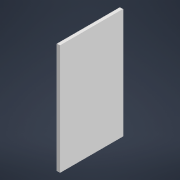
# Autodesk Inventor part: TorraumSeiteBalleinwurf
Saved by Autodesk Inventor 2021.4 (Build 254397000, 397)
## iProperties
Created: 2022-02-22
Part Number: TorraumSeiteBalleinwurf
Material: Generisch
Document SubType Name: Modeling
Designer: valen
Density: 1 g/cm^3
Appearance: Vorgabe
Author: valen
Autodesk Inventor part; units mm, degrees
ref_plane "YZ Plane" through (0, 0, 0) normal (1, 0, 0) x (0, 1, 0)
ref_plane "XZ Plane" through (0, 0, 0) normal (0, 1, 0) x (-1, 0, 0)
ref_plane "XY Plane" through (0, 0, 0) normal (0, 0, 1) x (1, 0, 0)
sketch "Skizze1" plane through (0, 0, 0) normal (1, 0, 0) x (0, 1, 0)
  line L0 (0, 0) -> (132, 0)
  line L1 (132, 0) -> (132, -80)
  line L2 (132, -80) -> (0, -80)
  line L3 (0, -80) -> (0, 0)
  dimension "d0" = 80
  dimension "d1" = 132
  constraints: 8 end point, 2 parallel, 1 horizontal, 1 perpendicular
  measures "d0" distance between parallel lines of L2 L0
  measures "d1" distance between parallel lines of L1 L3
extrude "Extrusion1" add sketch "Skizze1" along normal blind 4
sketch "Sketch2" plane through (0, 0, 0) normal (1, 0, 0) x (0, 1, 0)
  line L0 (0, 0) -> (0, -80) projected
  line L1 (0, 0) -> (-8, 0)
  line L2 (-8, 0) -> (-8, -80)
  line L3 (-8, -80) -> (0, -80)
  line L4 (0, -80) -> (0, 0)
  line L5 (0, -80) -> (132, -80) projected
  line L6 (132, 0) -> (0, 0) projected
  line L7 (132, 0) -> (0, 0) projected
  dimension "d5" = 8
  constraints: 8 end point, 2 collinear, 2 parallel, 1 horizontal, 1 perpendicular, 1 point on line
  measures "d5" distance between parallel lines of L2 L0
extrude "Extrusion2" add sketch "Sketch2" along normal blind 4
